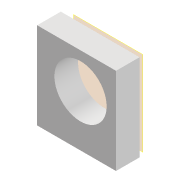
# Autodesk Inventor part: 30_Flexure_Laseradapter_XY
Saved by Autodesk Inventor 2022 (Build 260153000, 153)
## iProperties
Created: 2023-02-07
Part Number: 30_Flexure_Laseradapter_XY
Material: Generisch
Document SubType Name: Modeling
Designer: diederichbenedict
Density: 1 g/cm^3
Appearance: Vorgabe
Author: diederichbenedict
Autodesk Inventor part; units mm, degrees
ref_plane "YZ Plane" through (0, 0, 0) normal (1, 0, 0) x (0, 1, 0)
ref_plane "XZ Plane" through (0, 0, 0) normal (0, 1, 0) x (-1, 0, 0)
ref_plane "XY Plane" through (0, 0, 0) normal (0, 0, 1) x (1, 0, 0)
ref_plane "Arbeitsebene1" through (0, 0, 0) normal (0, 0, 1) x (1, 0, 0)
sketch "Skizze1" plane through (0, 0, 0) normal (0, 0, 1) x (1, 0, 0)
  line L0 (7.1, -14.0992) -> (0, -18.1984) projected
  line L1 (0, -18.1984) -> (-7.1, -14.0992) projected
  line L2 (-7.1, -14.0992) -> (-7.1, -5.9008) projected
  line L3 (-7.1, -5.9008) -> (0, -1.8016) projected
  line L4 (0, -1.8016) -> (7.1, -5.9008) projected
  line L5 (7.1, -5.9008) -> (7.1, -14.0992) projected
  line L6 (-8, -19.5) -> (8, -19.5) projected
  line L7 (8, 0) -> (8, -19.5) projected
  line L8 (-8, 0) -> (8, 0) projected
  line L9 (-8, -19.5) -> (-8, 0) projected
  line L10 (8, 0) -> (-12, 0)
  line L11 (-12, 0) -> (-12, -20)
  line L12 (-12, -20) -> (8, -20)
  line L13 (8, -20) -> (8, 0)
  circle A0 centre (-1, -9) radius 6.625
  circle A1 centre (0, -10) radius 6.5405 construction
  line L14 (-12, -20) -> (8, -20)
  line L15 (8, -20) -> (8, -22)
  line L16 (8, -22) -> (-12, -22)
  line L17 (-12, -22) -> (-12, -20)
  point P0 (0, 0)
  dimension "d0" = 20
  dimension "d1" = 20
  dimension "d2" = 13.25
  dimension "d4" = 1
  dimension "d7" = 20
  dimension "d8" = 2
  dimension "d9" = 1
  constraints: 16 end point, 4 parallel, 2 horizontal, 2 perpendicular, 1 centre point
  measures "d0" distance of L12.end L11.end
  measures "d1" distance of L11.end L10.end
  measures "d2" diameter of A0
  measures "d4" horizontal distance of A1.centre A0.centre
  measures "d7" distance of L15.end L16.end
  measures "d8" distance of L14.end L15.end
  measures "d9" horizontal distance of A0.centre A1.centre
extrude "Extrusion1" add sketch "Skizze1" along normal blind 6 contours L0 L1 L2 A0 L3 L4 L5 | L2 L3 A0 | L9 L8 L7 L6 | L6 L13 L12 L11 L10 L9 | L15 L16 L17 L12 picked at (-6.9868, -5.9999)
